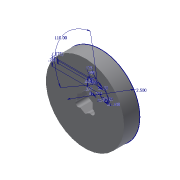
# Autodesk Inventor part: augmented gear v4
Saved by Autodesk Inventor 2014 (Build 180170000, 170)
## iProperties
Created: 2014-02-23
Part Number: augmented gear v4
Material: Generic
Document SubType Name: Modeling
Designer: Owner
Density: 1 g/cm^3
Appearance: Default
Author: Owner
Autodesk Inventor part; units mm, degrees
ref_plane "YZ Plane" through (0, 0, 0) normal (1, 0, 0) x (0, 1, 0)
ref_plane "XZ Plane" through (0, 0, 0) normal (0, 1, 0) x (-1, 0, 0)
ref_plane "XY Plane" through (0, 0, 0) normal (0, 0, 1) x (1, 0, 0)
sketch "Sketch1" plane through (0, 0, 0) normal (0, 0, 1) x (1, 0, 0)
  line L0 (0, 0) -> (0, 7.239) construction
  line L1 (0, 0) -> (6.2692, 3.6195) construction
  line L2 (0, 0) -> (6.2692, -3.6195) construction
  line L3 (0, 0) -> (0, -7.239) construction
  line L4 (0, 0) -> (-6.2692, -3.6195) construction
  line L5 (0, 0) -> (-6.2692, 3.6195) construction
  line L6 (0, 7.239) -> (6.2692, 3.6195)
  line L7 (6.2692, 3.6195) -> (6.2692, -3.6195)
  line L8 (6.2692, -3.6195) -> (0, -7.239)
  line L9 (0, -7.239) -> (-6.2692, -3.6195)
  line L10 (-6.2692, -3.6195) -> (-6.2692, 3.6195)
  line L11 (-6.2692, 3.6195) -> (0, 7.239)
  circle A0 centre (0, 0) radius 31.75
  line L12 (0, 0) -> (0, 6.4008)
  circle A1 centre (0, 6.4008) radius 2.3813
  circle A2 centre (0, 4.4894) radius 2.3813 construction
  line L13 (-2.9354, 9.3347) -> (-2.3293, 5.8974) construction
  line L14 (2.3813, 6.4008) -> (-2.3813, 6.4008)
  line L15 (2.3813, 6.4008) -> (2.3813, 5.8642)
  line L16 (-2.3813, 6.4008) -> (-2.3813, 5.8642)
  line L17 (2.3813, 5.8642) -> (-2.3813, 5.8642)
  line L18 (0, 0) -> (5.5433, -3.2004)
  line L19 (0, 0) -> (-5.5433, -3.2004)
  circle A3 centre (5.5433, -3.2004) radius 2.3813
  circle A4 centre (-5.5433, -3.2004) radius 2.2509
  line L20 (6.7339, -1.1382) -> (4.3526, -5.2626)
  line L21 (6.7339, -1.1382) -> (6.2692, -0.8699)
  line L22 (4.3526, -5.2626) -> (3.8879, -4.9943)
  line L23 (6.2692, -0.8699) -> (3.8879, -4.9943)
  line L24 (-6.6687, -1.2511) -> (-4.4178, -5.1497)
  line L25 (-4.4178, -5.1497) -> (-4.0183, -4.9191)
  line L26 (-6.6687, -1.2511) -> (-6.2692, -1.0204)
  line L27 (-6.2692, -1.0204) -> (-4.0183, -4.9191)
  dimension "d0" = 7.239
  dimension "d1" = 60
  dimension "d2" = 60
  dimension "d6" = 63.5
  dimension "d15" = 4.7625
  dimension "d16" = 6.4008
  dimension "d19" = 4.7625
  dimension "d22" = 110
  dimension "d23" = 4.551
  dimension "d24" = 3.4903
  dimension "d25" = 6.4008
  dimension "d26" = 6.4008
  dimension "d27" = 4.5018
  dimension "d28" = 4.7625
  dimension "d31" = 1.9114
  constraints: 56 end point, 13 equal length, 10 point on line, 8 tangent, 7 perpendicular, 6 point on circle, 5 centre point, 4 coincident, 3 line through centre, 1 vertical
  measures "d0" distance of L0.start L0.end
  measures "d1" angle of L0 L1
  measures "d2" angle of L2 L1
  measures "d6" diameter of A0
  measures "d15" diameter of A1
  measures "d16" distance of L12.start L12.end
  measures "d19" diameter of A2
  measures "d22" angle of L11 L13
  measures "d23" distance of L13.end L5.end
  measures "d24" distance of L13.start L13.end
  measures "d25" distance of L12.start L18.end
  measures "d26" distance of L12.start L19.end
  measures "d27" diameter of A4
  measures "d28" diameter of A3
  measures "d31" distance of L12.end A2.centre
extrude "Extrusion5" add sketch "Sketch1" along normal blind 12.7
equation "\"d25\" = d16"
equation "\"d26\" = d16"
equation "\"d28\" = d15"
body "Solid2"
